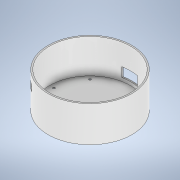
# Autodesk Inventor part: caseTop
Saved by Autodesk Inventor 2020 (Build 240168000, 168)
## iProperties
Created: 2020-04-07
Part Number: caseTop
Material: Пластик АБС
Document SubType Name: Modeling
Designer: jamnissa
Density: 1.06 g/cm^3
Appearance: Гладкий — белый
Mass: 57.326 g
Surface Area: 551.939 cm^2
Volume: 54.0811 cm^3
Author: jamnissa
Autodesk Inventor part; units mm, degrees
ref_plane "YZ Plane" through (0, 0, 0) normal (1, 0, 0) x (0, 1, 0)
ref_plane "XZ Plane" through (0, 0, 0) normal (0, 1, 0) x (-1, 0, 0)
ref_plane "XY Plane" through (0, 0, 0) normal (0, 0, 1) x (1, 0, 0)
sketch "Эскиз1" plane through (0, 0, 0) normal (0, 1, 0) x (-1, 0, 0)
  circle A0 centre (0, 0) radius 58
  line L0 (79.4555, 0) -> (-79.4555, 0)
  line L1 (0, -106.6382) -> (0, 90.6575)
  dimension "d0" = 116
  constraints: 4 end point, 1 centre point, 1 coincident, 1 horizontal, 1 midpoint, 1 point on line, 1 vertical
  measures "d0" diameter of A0
extrude "Выдавливание1" add sketch "Эскиз1" along normal blind 2
sketch "Эскиз2" plane through (0, 0, 0) normal (0, -1, 0) x (1, 0, 0)
  circle A0 centre (0, 0) radius 57
  line L0 (0, -103.8803) -> (0, 88.3129)
  line L1 (-79.4555, 0) -> (79.4555, 0) projected
  circle A1 centre (0, 0) radius 50
  circle A2 centre (0, -50) radius 1.5
  circle A3 centre (50, 0) radius 1.5
  circle A4 centre (0, 50) radius 1.5
  circle A5 centre (-50, 0) radius 1.5
  circle A6 centre (35.3553, -35.3553) radius 1.5
  circle A7 centre (50, 0) radius 1.5
  circle A8 centre (35.3553, 35.3553) radius 1.5
  circle A9 centre (0, 50) radius 1.5
  circle A10 centre (-35.3553, 35.3553) radius 1.5
  circle A11 centre (-50, 0) radius 1.5
  circle A12 centre (-35.3553, -35.3553) radius 1.5
  dimension "d22" = 3
  dimension "d23" = 3
  dimension "d26" = 3
  dimension "d30" = 360
  dimension "d84" = 114
  constraints: 13 centre point, 4 point on circle, 4 point on line, 2 end point, 1 coincident, 17 other
  measures "d22" diameter of A2
  measures "d23" diameter of A3
  measures "d26" diameter of A5
  measures "d84" diameter of A0
sketch "Эскиз6" plane through (0, 2, 0) normal (0, 1, 0) x (1, 0, 0)
  circle A0 centre (0, 0) radius 58 projected
  dimension "d85" = 116
  measures "d85" diameter of A0
ref_plane "РабПлоскость2" through (0, 49.211, 0) normal (0, 1, 0) x (1, 0, 0)
sketch "Эскиз7" plane through (0, 49.211, 0) normal (0, 1, 0) x (1, 0, 0)
  circle A0 centre (0, 0) radius 58 projected
  dimension "d86" = 116
  measures "d86" diameter of A0
loft "Лофт1" add profiles "Эскиз7", "Эскиз6"
sketch "Эскиз8" plane through (0, 49.211, 0) normal (0, 1, 0) x (1, 0, 0)
  circle A0 centre (0, 0) radius 56
  dimension "d83" = 112
  constraints: 1 centre point, 1 coincident
  measures "d83" diameter of A0
extrude "Выдавливание9" cut sketch "Эскиз8" against normal blind 47.211
ref_plane "РабПлоскость6" through (-79.4555, 0, 0) normal (0, 0, -1) x (1, 0, 0)
sketch "Эскиз10" plane through (-79.4555, 0, 0) normal (0, 0, -1) x (1, 0, 0)
  line L0 (137.4555, -49.211) -> (21.4555, -49.211) projected
  line L1 (79.4555, 0) -> (79.4555, -49.211)
  line L2 (68.4555, -6.6479) -> (90.4555, -6.6479)
  line L3 (90.4555, -6.6479) -> (90.4555, -19.6479)
  line L4 (90.4555, -19.6479) -> (68.4555, -19.6479)
  line L5 (68.4555, -19.6479) -> (68.4555, -6.6479)
  line L6 (60.4965, -15.4479) -> (98.4145, -15.4479)
  line L7 (98.4145, -15.4479) -> (98.4145, -23.8479)
  line L8 (98.4145, -23.8479) -> (60.4965, -23.8479)
  line L9 (60.4965, -23.8479) -> (60.4965, -15.4479)
  circle A0 centre (60.4965, -15.4479) radius 1.15
  circle A1 centre (98.4145, -15.4479) radius 1.15
  line L10 (45.8699, -29.3481) -> (39.8699, -29.3481)
  line L11 (39.8699, -29.3481) -> (39.8699, -37.3481)
  line L12 (39.8699, -37.3481) -> (45.8699, -37.3481)
  line L13 (45.8699, -37.3481) -> (45.8699, -29.3481)
  point P0 (79.4555, 0)
  dimension "d94" = 22
  dimension "d95" = 13
  dimension "d101" = 37.918
  dimension "d102" = 8.4
  dimension "d103" = 2.3
  dimension "d104" = 2.3
  dimension "d114" = 6
  dimension "d115" = 8
  constraints: 26 end point, 6 parallel, 3 horizontal, 3 perpendicular, 2 centre point, 2 coincident, 1 midpoint, 2 other
  measures "d94" distance of L2.start L2.end
  measures "d95" distance of L2.end L3.end
  measures "d101" distance of L6.start L6.end
  measures "d102" distance of L6.end L7.end
  measures "d103" diameter of A0
  measures "d104" diameter of A1
  measures "d114" distance of L12.end L11.end
  measures "d115" distance of L11.end L10.end
extrude "Выдавливание11" cut sketch "Эскиз10" along normal blind 60 contours L2 L3 L6 L1 | L1 L6 L5 L2 | L6 L3 L4 L1 | L1 L4 L5 L6
hole "Отверстие1" at (0, 0, 50) at (-35.3553, 0, 35.3553) at (35.3553, 0, 35.3553) at (50, 0, 0) at (35.3553, 0, -35.3553) at (-35.3553, 0, -35.3553) at (-50, 0, 0) direction (0, 1, 0) diameter 3 end through all countersink diameter 5.6 countersink angle 90
extrude "Выдавливание13" cut sketch "Эскиз10" against normal blind 60 contours L13 L12 L11 L10
